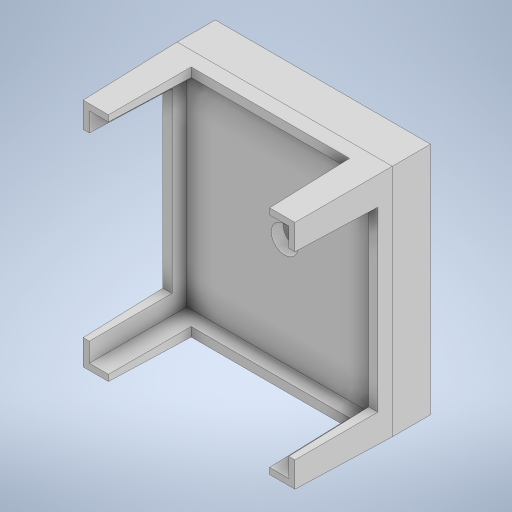
# Autodesk Inventor part: Część5
Saved by Autodesk Inventor 2024.3 (Build 283343000, 343)
## iProperties
Created: 2024-07-18
Part Number: Część5
Material: Ogólny
Document SubType Name: Modeling
Designer: User
Density: 1 g/cm^3
Appearance: Domyślna
Author: User
## iProperties of the stored document Część5_Drukowanie 3D.ipt
Created: 2024-07-20
Part Number: Część5_Drukowanie 3D
Material: Ogólny
Document SubType Name: Modeling
Designer: User
Density: 1 g/cm^3
Appearance: Domyślna
Author: User
Autodesk Inventor part; units mm, degrees
ref_plane "YZ Plane" through (0, 0, 0) normal (1, 0, 0) x (0, 1, 0)
ref_plane "XZ Plane" through (0, 0, 0) normal (0, 1, 0) x (-1, 0, 0)
sketch "Szkic1" plane through (0, 0, 0) normal (0, 0, 1) x (1, 0, 0)
  line L0 (0, 0) -> (41, 0)
  line L1 (41, 0) -> (41, 45)
  line L2 (41, 45) -> (0, 45)
  line L3 (0, 45) -> (0, 0)
  line L4 (0, 45) -> (-2, 45)
  line L5 (-2, 45) -> (-2, 47)
  line L6 (41, 0) -> (41, -2)
  line L7 (41, -2) -> (43, -2)
  line L8 (43, -2) -> (-2, -2)
  line L9 (-2, -2) -> (-2, 47)
  line L10 (-2, 47) -> (43, 47)
  line L11 (43, 47) -> (43, -2)
  line L12 (41, 45) -> (37, 45)
  line L13 (37, 45) -> (37, 47)
  line L14 (43, 47) -> (37, 47)
  line L15 (41, 45) -> (41, 41)
  line L16 (41, 41) -> (43, 41)
  line L17 (43, 47) -> (43, 41)
  line L18 (43, 47) -> (37, 47)
  line L19 (20.5, 47) -> (20.5, -2)
  line L20 (-2, 22.5) -> (43, 22.5)
  line L21 (0, 45) -> (41, 45)
  line L22 (43, 47) -> (-2, 47)
  line L23 (-2, 47) -> (-2, -2)
  line L24 (4, 45) -> (4, 47)
  line L25 (0, 41) -> (-2, 41)
  line L26 (41, 0) -> (0, 0)
  line L27 (0, 0) -> (0, 45)
  line L28 (0, 0) -> (-2, 0)
  line L29 (-2, -2) -> (43, -2)
  line L30 (43, -2) -> (43, 47)
  line L31 (41, 4) -> (43, 4)
  line L32 (-2, -2) -> (-2, 47)
  line L33 (4, 0) -> (4, -2)
  line L34 (0, 0) -> (0, 4)
  line L35 (0, 4) -> (-2, 4)
  line L36 (41, 0) -> (37, 0)
  line L37 (37, 0) -> (37, -2)
  line L38 (37, -2) -> (43, -2)
  dimension "d0" = 41
  dimension "d1" = 45
  dimension "d2" = 2
  dimension "d3" = 2
  dimension "d4" = 2
  dimension "d5" = 2
  dimension "d6" = 4
  dimension "d7" = 4
  dimension "d8" = 4
  dimension "d9" = 4
  constraints: 78 end point, 21 symmetric about line, 12 point on line, 9 perpendicular, 4 midpoint, 4 parallel, 3 collinear, 3 horizontal, 1 vertical
  measures "d0" distance of L2.end L1.end
  measures "d1" distance of L1.end L0.end
  measures "d2" distance of L2.end L4.end
  measures "d3" distance of L4.end L5.end
  measures "d4" distance of L0.end L6.end
  measures "d5" distance of L6.end L7.end
  measures "d6" distance of L1.end L12.end
  measures "d7" distance of L1.end L15.end
  measures "d8" distance of L27.start L34.end
  measures "d9" distance of L26.start L36.end
sketch "Szkic1 outline for Wyciągnięcie proste1" plane through (0, 0, 0) normal (0, 0, 1) x (1, 0, 0)
  line L0 (41, 41) -> (43, 41)
  line L1 (41, 45) -> (41, 41)
  line L2 (37, 45) -> (41, 45)
  line L3 (37, 47) -> (37, 45)
  line L4 (43, 47) -> (37, 47)
  line L5 (43, 41) -> (43, 47)
  line L6 (43, 4) -> (41, 4)
  line L7 (41, 4) -> (41, 0)
  line L8 (41, 0) -> (37, 0)
  line L9 (37, 0) -> (37, -2)
  line L10 (37, -2) -> (43, -2)
  line L11 (43, -2) -> (43, 4)
  line L12 (0, 4) -> (-2, 4)
  line L13 (0, 0) -> (0, 4)
  line L14 (4, 0) -> (0, 0)
  line L15 (4, -2) -> (4, 0)
  line L16 (-2, -2) -> (4, -2)
  line L17 (-2, 4) -> (-2, -2)
  line L18 (4, 45) -> (4, 47)
  line L19 (4, 47) -> (-2, 47)
  line L20 (-2, 47) -> (-2, 41)
  line L21 (-2, 41) -> (0, 41)
  line L22 (0, 41) -> (0, 45)
  line L23 (0, 45) -> (4, 45)
extrude "Wyciągnięcie proste1" add sketch "Szkic1 outline for Wyciągnięcie proste1" along normal blind 20 draft -1
sketch "Szkic2" plane through (0, 0, 0) normal (0, 0, -1) x (-1, 0, 0)
  line L0 (-43, 41) -> (-43, 47) projected
  line L1 (2, 4) -> (2, -2) projected
  line L2 (-43, 47) -> (2, 47)
  line L3 (2, 47) -> (2, -2)
  line L4 (2, -2) -> (-43, -2)
  line L5 (-43, -2) -> (-43, 47)
  line L6 (-37, 45) -> (-41, 45) projected
  line L7 (0, 0) -> (-41, 0)
  line L8 (-41, 0) -> (-41, 45)
  line L9 (-41, 45) -> (0, 45)
  line L10 (0, 45) -> (0, 0)
  constraints: 16 end point, 4 parallel, 2 horizontal, 2 perpendicular
extrude "Wyciągnięcie proste2" add sketch "Szkic2" against normal blind 3 draft -1
sketch "Szkic3" plane through (0, 0, 0) normal (0, 0, -1) x (-1, 0, 0)
  line L0 (2, -2) -> (1.650899, -1.650899)
  line L1 (-43, -2) -> (-43, 47)
  line L2 (2, -2) -> (-43, -2)
  line L3 (-43, -2) -> (-43, 47)
  line L4 (-43, 47) -> (2, 47)
  line L5 (2, 47) -> (2, -2)
  circle A0 centre (-20.5, 22.5) radius 2.85
  circle A1 centre (-20.5, 22.5) radius 2.8
  point P0 (0, 0)
  dimension "d14" = 5.7
  dimension "d21" = 5.6
  constraints: 8 end point, 2 centre point, 2 parallel, 1 coincident, 1 horizontal, 1 perpendicular
  measures "d14" diameter of A0
  measures "d21" diameter of A1
extrude "Wyciągnięcie proste3" add sketch "Szkic3" along normal blind 8 contours L1 L4 L5 L2 | A0
ref_plane "Płaszczyzna konstrukcyjna2" through (43, 47, -4.5) normal (0, 0, -1) x (-1, 0, 0)
ref_plane "Płaszczyzna konstrukcyjna1" through (43, 47, -8) normal (0, 0, -1) x (-1, 0, 0)
sketch "Szkic4" plane through (43, 47, -4.5) normal (0, 0, -1) x (-1, 0, 0)
  circle A0 centre (22.5, -24.5) radius 2.85 projected
  circle A1 centre (22.5, -24.5) radius 1.5
  circle A2 centre (22.5, -24.5) radius 2.85
  point P0 (43, -47)
  dimension "d18" = 3
  constraints: 2 centre point, 2 coincident
  measures "d18" diameter of A1
extrude "Wyciągnięcie proste4" add sketch "Szkic4" along normal blind 1
sketch "Szkic5" plane through (20.5, 22.5, -5.5) normal (0, 0, -1) x (-1, 0, 0)
  circle A0 centre (0, 0) radius 2.8
  circle A1 centre (0, 0) radius 2.4
  point P0 (20.5, -22.5)
  dimension "d22" = 4.8
  constraints: 2 centre point, 1 coincident
  measures "d22" diameter of A1
extrude "Wyciągnięcie proste5" add sketch "Szkic5" along normal blind 2.5
sketch "Szkic6" plane through (20.5, 22.5, -4.5) normal (0, 0, 1) x (1, 0, 0)
  circle A0 centre (0, 0) radius 1.5
  circle A1 centre (0, 0) radius 2.8
  point P0 (-20.5, -22.5)
  constraints: 2 centre point, 1 coincident
extrude "Wyciągnięcie proste6" add sketch "Szkic6" along normal blind 2
sketch "Szkic7" plane through (20.5, 22.5, -5.5) normal (0, 0, -1) x (-1, 0, 0)
  circle A0 centre (0, 0) radius 1.5
  circle A1 centre (0, 0) radius 2.4
  point P0 (20.5, -22.5)
  constraints: 2 centre point, 1 coincident
extrude "Wyciągnięcie proste7" cut sketch "Szkic7" against normal blind 1.5
sketch "Szkic8" plane through (20.5, 22.5, -2.5) normal (0, 0, 1) x (1, 0, 0)
  circle A0 centre (0, 0) radius 1.4
  circle A1 centre (0, 0) radius 1.5
  point P0 (-20.5, -22.5)
  dimension "d29" = 2.8
  constraints: 2 centre point, 1 coincident
  measures "d29" diameter of A0
extrude "Wyciągnięcie proste8" add sketch "Szkic8" against normal blind 1.5
